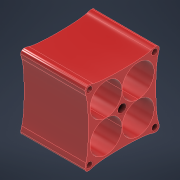
# Autodesk Inventor part: BatteryHolder
Saved by Autodesk Inventor 2022 (Build 260153000, 153)
## iProperties
Created: 2022-04-11
Part Number: BatteryHolder
Material: ABS Plastic
Document SubType Name: Modeling
Designer: ForseFire
Density: 1.06 g/cm^3
Appearance: Red
Author: ForseFire
Autodesk Inventor part; units mm, degrees
ref_plane "YZ Plane" through (0, 0, 0) normal (1, 0, 0) x (0, 1, 0)
ref_plane "XZ Plane" through (0, 0, 0) normal (0, 1, 0) x (-1, 0, 0)
ref_plane "XY Plane" through (0, 0, 0) normal (0, 0, 1) x (1, 0, 0)
sketch "Sketch1" plane through (0, 0, 0) normal (1, 0, 0) x (0, 1, 0)
  line L0 (-22, -22) -> (22, -22)
  line L1 (22, -22) -> (22, 22)
  line L2 (22, 22) -> (-22, 22)
  line L3 (-22, 22) -> (-22, -22)
  line L4 (-22, -22) -> (22, 22) construction
  line L5 (22, -22) -> (-22, 22) construction
  line L6 (-19.3, -19.3) -> (19.3, -19.3)
  line L7 (19.3, -19.3) -> (19.3, 19.3)
  line L8 (19.3, 19.3) -> (-19.3, 19.3)
  line L9 (-19.3, 19.3) -> (-19.3, -19.3)
  line L10 (-19.3, -19.3) -> (19.3, 19.3) construction
  line L11 (19.3, -19.3) -> (-19.3, 19.3) construction
  circle A0 centre (19.3, 19.3) radius 1.725
  circle A1 centre (19.3, -19.3) radius 1.725
  circle A2 centre (-19.3, -19.3) radius 1.725
  circle A3 centre (-19.3, 19.3) radius 1.725
  circle A4 centre (9.5, 9.5) radius 9.5
  circle A5 centre (9.5, -9.5) radius 9.5
  circle A6 centre (-9.5, -9.5) radius 9.5
  circle A7 centre (-9.5, 9.5) radius 9.5
  point P0 (0, 0)
  point P1 (0, 0)
  point P2 (0, 0)
  point P3 (-9.5, 0)
  point P4 (0, 9.5)
  point P5 (9.5, 0)
  point P6 (0, -9.5)
  dimension "d4" = 44
  dimension "d5" = 44
  dimension "d6" = 38.6
  dimension "d7" = 3.45
  dimension "d8" = 3.45
  dimension "d9" = 3.45
  dimension "d10" = 3.45
  dimension "d24" = 19
  dimension "d25" = 19
  dimension "d26" = 19
  dimension "d27" = 19
  constraints: 24 end point, 8 centre point, 6 midpoint, 5 point on line, 4 coincident, 4 parallel, 2 horizontal, 2 horizontal alignment, 2 perpendicular, 2 vertical alignment, 1 equal radius
  measures "d4" distance of L2.end L1.end
  measures "d5" distance of L0.end L1.end
  measures "d6" distance of L6.end L7.end
  measures "d7" diameter of A0
  measures "d8" diameter of A1
  measures "d9" diameter of A2
  measures "d10" diameter of A3
  measures "d24" diameter of A4
  measures "d25" diameter of A5
  measures "d26" diameter of A6
  measures "d27" diameter of A7
extrude "Extrusion1" add sketch "Sketch1" along normal blind 35 contours L3 L2 L1 L0 | A2 L9 A3 L8 A0 L7 A1 L6 | A4 A5 A6 A7
fillet "Fillet1" radius 2 4 edges at (17.5, -22, 22) (17.5, -22, -22) (17.5, 22, 22) (17.5, 22, -22)
sketch "Sketch3" plane through (0, 0, 0) normal (-1, 0, 0) x (0, 0, 1)
  circle A0 centre (19.3, 19.3) radius 1.725 projected
  arc A1 (0, -9.5) -> (9.5, 0) centre (9.5, -9.5) ccw projected
  arc A2 (-9.5, 0) -> (0, -9.5) centre (-9.5, -9.5) ccw projected
  arc A3 (0, 9.5) -> (-9.5, 0) centre (-9.5, 9.5) ccw projected
  arc A4 (9.5, 0) -> (0, 9.5) centre (9.5, 9.5) ccw projected
  circle A5 centre (-19.3, 19.3) radius 1.725 projected
  circle A6 centre (-19.3, -19.3) radius 1.725 projected
  circle A7 centre (19.3, -19.3) radius 1.725 projected
  arc A8 (22, 20) -> (20, 22) centre (20, 20) ccw projected
  line L0 (-20, 22) -> (20, 22) projected
  line L1 (-22, -20) -> (-22, 20) projected
  arc A9 (-22, -20) -> (-20, -22) centre (-20, -20) ccw projected
  line L2 (20, -22) -> (-20, -22) projected
  arc A10 (20, -22) -> (22, -20) centre (20, -20) ccw projected
  line L3 (22, 20) -> (22, -20) projected
  circle A11 centre (9.5, -9.5) radius 5
  circle A12 centre (-9.5, -9.5) radius 5
  circle A13 centre (-9.5, 9.5) radius 5
  circle A14 centre (9.5, 9.5) radius 5
  arc A15 (-20, 22) -> (-22, 20) centre (-20, 20) ccw projected
  point P0 (0, 0)
  dimension "d28" = 10
  dimension "d29" = 10
  dimension "d30" = 10
  dimension "d31" = 10
  constraints: 4 centre point, 4 coincident
  measures "d28" diameter of A11
  measures "d29" diameter of A12
  measures "d30" diameter of A13
  measures "d31" diameter of A14
extrude "Extrusion3" add sketch "Sketch3" along normal blind 3 contours A2 A3 A4 A1 | L3 A10 L2 A9 L1 A15 L0 A8
sketch "Sketch4" plane through (35, 0, 0) normal (1, 0, 0) x (0, 0, -1)
  arc A0 (9.5, 0) -> (0, -9.5) centre (9.5, -9.5) ccw projected
  arc A1 (0, 9.5) -> (9.5, 0) centre (9.5, 9.5) ccw projected
  arc A2 (-9.5, 0) -> (0, 9.5) centre (-9.5, 9.5) ccw projected
  arc A3 (0, -9.5) -> (-9.5, 0) centre (-9.5, -9.5) ccw projected
  circle A4 centre (0, 0) radius 2.5
  dimension "d34" = 5
  constraints: 1 centre point, 1 coincident
  measures "d34" diameter of A4
extrude "Extrusion4" cut sketch "Sketch4" against normal blind 38 contours A4
sketch "Sketch10" plane through (35, 0, 0) normal (1, 0, 0) x (0, 0, -1)
  line L0 (-20, -22) -> (20, -22) projected
  ellipse E0 centre (0, -22) end of major axis (-18, -22) minor radius 2
  line L1 (22, -20) -> (22, 20) projected
  ellipse E1 centre (22, 0) end of major axis (22, 18) minor radius 2
  line L2 (20, 22) -> (-20, 22) projected
  ellipse E2 centre (0, 22) end of major axis (-18, 22) minor radius 2
  line L3 (-22, 20) -> (-22, -20) projected
  ellipse E3 centre (-22, 0) end of major axis (-22, 18) minor radius 2
  point P0 (0, 0)
  dimension "d47" = 18
  dimension "d48" = 2
  dimension "d49" = 2
  dimension "d50" = 18
  dimension "d51" = 2
  dimension "d52" = 18
  dimension "d53" = 2
  dimension "d54" = 18
  constraints: 4 midpoint, 8 other
extrude "Extrusion8" cut sketch "Sketch10" against normal blind 38
fillet "Fillet2" radius 10 8 edges at (16, 22, -18) (16, 18, -22) (16, 22, 18) (16, 18, 22) (16, -18, -22) (16, -22, -18) (16, -22, 18) (16, -18, 22)
body "Solid1"
